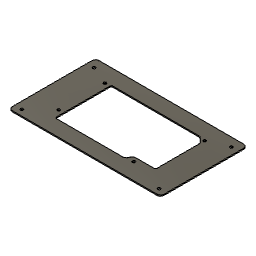
XT ATX Bracket (Autodesk Fusion 360 design; units mm, degrees)
Autodesk Fusion 360 part; units mm, degrees
note: some values were not read from the file. Set by a fixed rule: which sketch regions a step uses.
sketch "XT ATX Bracket Sketch" plane through (0, 0, 0) normal (0, 0, 1) x (1, 0, 0)
  line L0 (100, 60) -> (-100, 60)
  line L1 (-105, 55) -> (-105, -55)
  line L2 (-100, -60) -> (100, -60)
  line L3 (105, -55) -> (105, 55)
  line L4 (105, 60) -> (-105, -60) construction
  line L5 (-105, 60) -> (105, -60) construction
  line L6 (-105, 48) -> (105, 48) construction
  line L7 (-105, -52) -> (105, -52) construction
  line L8 (95, 60) -> (95, -60) construction
  line L9 (-95, 60) -> (-95, -60) construction
  circle A0 centre (-95, 48) radius 2
  circle A1 centre (95, 48) radius 2
  circle A2 centre (95, -52) radius 2
  circle A3 centre (-95, -52) radius 2
  line L10 (75, 43) -> (-75, 43)
  line L11 (-75, 43) -> (-75, -43)
  line L12 (-75, -43) -> (75, -43)
  line L13 (75, -43) -> (75, 43)
  line L14 (75, 43) -> (-75, -43) construction
  line L15 (-75, 43) -> (75, -43) construction
  line L16 (-69, 43) -> (-69, -43) construction
  line L17 (-75, 37) -> (75, 37) construction
  line L18 (69, 37) -> (69, 43) construction
  line L19 (45, -37) -> (75, -37) construction
  line L20 (45, -37) -> (45, -43) construction
  line L21 (-69, -27) -> (-75, -27) construction
  circle A4 centre (-69, 37) radius 2
  circle A5 centre (69, 37) radius 2
  circle A6 centre (-69, -27) radius 2
  circle A7 centre (45, -37) radius 2
  line L22 (-62, 39) -> (-62, -39)
  line L23 (-62, -39) -> (34.4133, -39)
  line L24 (34.4133, -39) -> (39, -31)
  line L25 (39, -31) -> (69, -31)
  line L26 (69, -31) -> (69, 39)
  line L27 (69, 39) -> (-62, 39)
  line L28 (75, 43) -> (65, 43) construction
  line L29 (65, 43) -> (65, 35) construction
  line L30 (65, 35) -> (75, 35) construction
  line L31 (75, 35) -> (75, 43) construction
  line L32 (65, 35) -> (69, 31)
  line L33 (65, 35) -> (61, 39)
  arc A8 (-100, 60) -> (-105, 55) centre (-100, 55) ccw
  arc A9 (105, 55) -> (100, 60) centre (100, 55) ccw
  arc A10 (100, -60) -> (105, -55) centre (100, -55) ccw
  arc A11 (-105, -55) -> (-100, -60) centre (-100, -55) ccw
  line L34 (42, 30) -> (66, 30) construction
  line L35 (66, 30) -> (66, 6) construction
  line L36 (66, 6) -> (42, 6) construction
  line L37 (42, 6) -> (42, 30) construction
  line L38 (66, 30) -> (68, 32) construction
  point P0 (-95, 48)
  point P1 (95, 48)
  point P2 (95, -52)
  point P3 (-95, -52)
  point P4 (-69, 37)
  point P5 (45, -37)
  point P6 (-69, -27)
  point P7 (69, 37)
  dimension "d11" = 210
  dimension "d14" = 120
  dimension "d15" = 12
  dimension "d16" = 8
  dimension "d28" = 10
  dimension "d31" = 10
  dimension "d33" = 4
  dimension "d34" = 150
  dimension "d35" = 86
  dimension "d41" = 6
  dimension "d43" = 6
  dimension "d46" = 16
  dimension "d47" = 6
  dimension "d48" = 30
  dimension "d49" = 6
  dimension "d51" = 4
  dimension "d52" = 64
  dimension "d53" = 114
  dimension "d54" = 74
  dimension "d55" = 138
  dimension "d62" = 13
  dimension "d63" = 4
  dimension "d64" = 6
  dimension "d65" = 4
  dimension "d66" = 12
  dimension "d67" = 36
  dimension "d72" = 10
  dimension "d73" = 8
  dimension "d74" = 5
  dimension "d98" = 24
  dimension "d99" = 24
  dimension "d100" = 9
  dimension "d101" = 13
  dimension "d102" = 2.8284
  constraint horizontal L0
  constraint perpendicular L0 L1
  constraint parallel L0 L2
  constraint coincident L1 L6.start
  constraint coincident L3 L6.end
  constraint perpendicular L3 L6
  constraint coincident L1 L7.start
  constraint midpoint L5 origin
  constraint coincident L3 L7.end
  constraint coincident L0 L8.start
  constraint coincident L2 L8.end
  constraint perpendicular L2 L8
  constraint coincident L0 L9.start
  constraint coincident L2 L9.end
  constraint perpendicular L2 L9
  constraint coincident L9 P0
  constraint coincident L6 P0
  constraint coincident L6 P1
  constraint coincident L8 P1
  constraint coincident L7 P2
  constraint coincident L8 P2
  constraint coincident L9 P3
  constraint coincident L7 P3
  constraint coincident P0 A0.centre
  constraint coincident P1 A1.centre
  constraint coincident P2 A2.centre
  constraint coincident P3 A3.centre
  constraint equal A0 A1
  constraint equal A1 A2
  constraint equal A2 A3
  constraint horizontal L10
  constraint perpendicular L10 L11
  constraint parallel L10 L12
  constraint parallel L11 L13
  constraint coincident L14 origin
  constraint coincident L15 origin
  constraint coincident L10 L16.start
  constraint coincident L12 L16.end
  constraint perpendicular L12 L16
  constraint coincident L11 L17.start
  constraint coincident L13 L17.end
  constraint perpendicular L13 L17
  constraint coincident L16 P4
  constraint coincident L17 P4
  constraint coincident L16 P6
  constraint coincident L17 P7
  constraint coincident P7 L18.start
  constraint coincident L10 L18.end
  constraint perpendicular L10 L18
  constraint coincident P5 L19.start
  constraint coincident L13 L19.end
  constraint perpendicular L13 L19
  constraint coincident L12 L20.end
  constraint perpendicular L12 L20
  constraint coincident P6 L21.start
  constraint coincident L11 L21.end
  constraint perpendicular L11 L21
  constraint coincident P4 A4.centre
  constraint equal A4 A5
  constraint equal A5 A7
  constraint equal A6 A7
  constraint perpendicular L6 L22
  constraint perpendicular L22 L23
  constraint perpendicular L15 L24
  constraint parallel L23 L25
  constraint perpendicular L25 L26
  constraint perpendicular L22 L27
  constraint horizontal L28
  constraint vertical L29
  constraint horizontal L30
  constraint vertical L31
  constraint coincident L26 L32.end
  constraint coincident L27 L33.end
  constraint collinear L32 L33
  constraint equal L32 L33
  constraint coincident L5.start L1
  constraint coincident L5.start L0
  constraint tangent L1 A8
  constraint tangent L0 A8
  constraint coincident L4.start L0
  constraint coincident L4.start L3
  constraint tangent L0 A9
  constraint tangent L3 A9
  constraint coincident L5.end L3
  constraint coincident L5.end L2
  constraint tangent L3 A10
  constraint tangent L2 A10
  constraint equal A9 A10
  constraint coincident L4.end L2
  constraint coincident L4.end L1
  constraint tangent L2 A11
  constraint tangent L1 A11
  constraint equal A9 A11
  constraint equal A8 A11
  constraint horizontal L34
  constraint vertical L35
  constraint horizontal L36
  constraint vertical L37
  constraint coincident L32 L38.end
  constraint perpendicular L32 L38
  measures "d11" distance of L4.end L5.end
  measures "d14" distance of L5.start L4.end
  measures "d15" distance of L0 L6
  measures "d16" distance of L2 L7
  measures "d28" distance of L1 L9
  measures "d31" distance of L3 L8
  measures "d33" diameter of A0
  measures "d34" distance of L11.end L12.end
  measures "d35" distance of L10.end L11.end
  measures "d41" distance of L10 L17
  measures "d43" distance of L11 L16
  measures "d46" distance of L12 L21
  measures "d47" distance of P5 L20.end
  measures "d48" distance of P5 L19.end
  measures "d49" distance of L13 L18
  measures "d51" diameter of A4
  measures "d52" distance of P4 P6
  measures "d53" horizontal distance of P5 P6
  measures "d54" vertical distance of P5 P7
  measures "d55" distance of P4 P7
  measures "d62" distance of L11 L22
  measures "d63" distance of L10 L27
  measures "d64" distance of L13 L26
  measures "d65" distance of L12 L23
  measures "d66" distance of L12 L25
  measures "d67" distance of L13 L24.end
  measures "d72" distance of L10.start L28.end
  measures "d73" distance of L10.start L30.end
  measures "d74" radius of A8
  measures "d98" distance of L34.start L34.end
  measures "d99" distance of L34.start L36.end
  measures "d100" distance of L13 L35
  measures "d101" distance of L10 L34
  measures "d102" distance of L34.end L38.end
extrude "Face1" add sketch "XT ATX Bracket Sketch" sketch "XT ATX Bracket Sketch" sketch "XT ATX Bracket Sketch" along normal blind 1.4986 contours L0 L1 L2 L3 A8 A9 A10 A11 of sketch 2 contours L0 L1 L2 L3 A8 A9 A10 A11 | L10 L11 L12 L13 of sketch 3 contours L0 L1 L2 L3 A8 A9 A10 A11 | L10 L11 L12 L13 | A5 L26 L27 L32 L33
fillet "Fillet1" radius 5 1 edges at (39, -31, 0.7493)
fillet "Fillet1" radius 2 3 edges at (-62, -39, 0.7493) (-62, 39, 0.7493) (69, -31, 0.7493)
fillet "Fillet1" radius 5 3 edges at (34.4133, -39, 0.7493) (61, 39, 0.7493) (69, 31, 0.7493)
equation "XTScrewTopOffset = 12 mm"
equation "XTScrewBottomOffset = 8 mm"
equation "d11 = XTWidth"
equation "d14 = XTHeight"
equation "d15 = XTScrewTopOffset"
equation "d16 = XTScrewBottomOffset"
equation "XTWidth = 210 mm"
equation "XTHeight = 120 mm"
equation "ATXWidth = 150 mm"
equation "ATXHeight = 86 mm"
equation "d28 = XTScrewLeftOffset"
equation "XTScrewLeftOffset = 10 mm"
equation "XTScrewRightOffset = 10 mm"
equation "d31 = XTScrewRightOffset"
equation "XTMountingHoleDiameter = 4 mm"
equation "d33 = XTMountingHoleDiameter"
equation "d34 = ATXWidth"
equation "d35 = ATXHeight"
equation "ATXScrewBottomOffsetLeft = 16 mm"
equation "ATXScrewTopOffset = 6 mm"
equation "ATXScrewRightOffsetTop = 6 mm"
equation "ATXScrewLeftOffset = 6 mm"
equation "d41 = ATXScrewTopOffset"
equation "d43 = ATXScrewLeftOffset"
equation "ATXScrewRightOffsetBottom = 30 mm"
equation "ATXScrewBottomOffsetRight = 6 mm"
equation "d46 = ATXScrewBottomOffsetLeft"
equation "d47 = ATXScrewBottomOffsetRight"
equation "d48 = ATXScrewRightOffsetBottom"
equation "d49 = ATXScrewRightOffsetTop"
equation "ATXMountingHoleDiameter = 4 mm"
equation "d51 = ATXMountingHoleDiameter"
equation "TopMountingGap = 5 mm - FeatureGap"
equation "LeftMountingGap = 14 mm - FeatureGap"
equation "RightMountingGap = 7 mm - FeatureGap"
equation "BottomMountingGap = TopMountingGap"
equation "BottomMountingGapRight = 13 mm - FeatureGap"
equation "RightMountingGapBottom = ATXScrewRightOffsetBottom + 6 mm"
equation "d62 = LeftMountingGap"
equation "d63 = TopMountingGap"
equation "d64 = RightMountingGap"
equation "d65 = BottomMountingGap"
equation "d66 = BottomMountingGapRight"
equation "d67 = RightMountingGapBottom"
equation "FeatureGap = 1 mm"
equation "ATXTopRightExtra = LeftMountingGap - ATXScrewLeftOffset"
equation "ATXTopRightExtraHeight = TopMountingGap + ATXMountingHoleDiameter"
equation "ATXTopRightExtraWidth = RightMountingGap + ATXMountingHoleDiameter"
equation "d72 = ATXTopRightExtraWidth"
equation "d73 = ATXTopRightExtraHeight"
equation "d74 = OutsideFillet"
equation "OutsideFillet = 5 mm"
equation "d78 = OutsideFillet"
equation "d90 = Inside90Fillet"
equation "Inside90Fillet = 2 mm"
equation "Inside45Fillet = 5 mm"
equation "d94 = Inside45Fillet"
equation "SwitchHeight = 24 mm"
equation "SwitchOffsetTop = 13 mm"
equation "SwitchOffsetRight = 9 mm"
equation "d98 = SwitchHeight"
equation "d99 = SwitchHeight"
equation "d100 = SwitchOffsetRight"
equation "d101 = SwitchOffsetTop"
